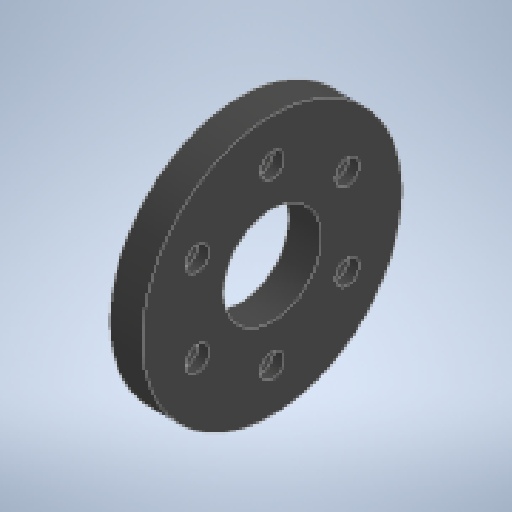
# Autodesk Inventor part: Spacer 3-8x .125
Saved by Autodesk Inventor 2023.2 (Build 272271000, 271)
## iProperties
Created: 2021-12-12
Part Number: Spacer 3-8x .125
Material: UHMW, Black
Document SubType Name: Modeling
Designer: NCai2
Density: 0.94 g/cm^3
Appearance: Rubber - Black
Mass: 2.24924 g
Surface Area: 25.3188 cm^2
Volume: 2.39281 cm^3
Author: NCai2
Autodesk Inventor part; units mm, degrees
ref_plane "YZ Plane" through (0, 0, 0) normal (1, 0, 0) x (0, 1, 0)
ref_plane "XZ Plane" through (0, 0, 0) normal (0, 1, 0) x (-1, 0, 0)
ref_plane "XY Plane" through (0, 0, 0) normal (0, 0, 1) x (1, 0, 0)
sketch "Sketch1" plane through (0, 0, 0) normal (1, 0, 0) x (0, 1, 0)
  circle A0 centre (0, 0) radius 7.1437
  circle A1 centre (0, 0) radius 19.05
  circle A2 centre (12.7, 0) radius 1.7526
  circle A3 centre (6.35, 10.9985) radius 1.7526
  circle A4 centre (-6.35, 10.9985) radius 1.7526
  circle A5 centre (-12.7, 0) radius 1.7526
  circle A6 centre (-6.35, -10.9985) radius 1.7526
  circle A7 centre (6.35, -10.9985) radius 1.7526
  dimension "d0" = 14.2875
  dimension "d1" = 38.1
  dimension "d4" = 3.5052
  dimension "d5" = 12.7
  dimension "d8" = 360
  constraints: 8 centre point, 2 coincident, 13 other
  measures "d0" diameter of A0
  measures "d1" diameter of A1
  measures "d4" diameter of A2
  measures "d5" distance of point (0, 0) A2.centre
extrude "Extrusion1" add sketch "Sketch1" along normal blind 4.7625
chamfer "Chamfer1" distance 3.175 angle 45 6 edges at (0, 10.9474, 0) (0, 4.5974, 10.9985) (0, -14.4526, 0) (0, -8.1026, 10.9985) (0, 4.5974, -10.9985) (0, -8.1026, -10.9985)
body "Solid1"
